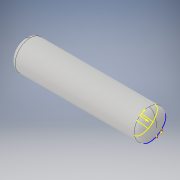
# Autodesk Inventor part: ModeloVaso
Saved by Autodesk Inventor 2019 (Build 230136000, 136)
## iProperties
Created: 2018-09-09
Part Number: ModeloVaso
Material: Generic
Document SubType Name: Modeling
Designer: leona
Density: 1 g/cm^3
Appearance: Default
Author: leona
Autodesk Inventor part; units mm, degrees
ref_plane "XZ Plane" through (0, 0, 0) normal (0, 1, 0) x (-1, 0, 0)
sketch "Sketch1" plane through (0, 0, 0) normal (0, 0, 1) x (1, 0, 0)
  line L0 (0, 50) -> (0, 0) construction
  line L1 (0, 0) -> (200, 0)
  line L2 (0, 50) -> (200, 50)
  ellipse E0 centre (200, 0) end of major axis (200, 50) minor radius 25 (225, 0) -> (200, 50) ccw
  line L3 (200, 0) -> (225, 0)
  line L4 (0, 50) -> (0, 0)
  line L5 (225, 0) -> (0, 0)
  dimension "d2" = 25
  dimension "d0" = 50
  dimension "d1" = 200
  constraints: 12 end point, 3 horizontal, 2 perpendicular, 1 coincident, 1 collinear, 1 point on line, 1 vertical, 4 other
  measures "d0" distance of L0.start L0.end
  measures "d1" distance of L0.end L1.end
revolve "Revolution1" add sketch "Sketch1" angle 360 about axis through (0, 0, 0) along (1, 0, 0)
mirror "Mirror1" about plane through (0, 50, 0) normal (-1, 0, 0) of "Revolution1"
ref_plane "Work Plane3" through (225, 0, 0) normal (1, 0, 0) x (0, 1, 0)
sketch "Sketch4" plane through (225, 0, 0) normal (1, 0, 0) x (0, 1, 0)
  line L0 (0, 0) -> (0, -20)
  line L1 (0, -20) -> (-1, -20)
  line L2 (1, -20) -> (0, -20)
  line L3 (1, -20) -> (0, -25)
  line L4 (0, -25) -> (-1, -20)
  line L5 (-20, 0) -> (-20, 1)
  line L6 (-20, -1) -> (-20, 0)
  line L7 (-20, -1) -> (-25, 0)
  line L8 (-25, 0) -> (-20, 1)
  line L9 (0, 0) -> (-20, 0)
  line L10 (0, 0) -> (50, 0) projected
  line L11 (-45.6527, 20.3919) -> (9.5558, -49.0784)
  circle A0 centre (0, 0) radius 50 projected
  line L12 (-18.0485, -14.3432) -> (0, 0)
  point P0 (-14.5002, -18.8081)
  point P1 (-26.6139, -3.5651)
  dimension "d6" = 1
  dimension "d13" = 5
  dimension "d14" = 20
  dimension "d17" = 90
  constraints: 24 end point, 4 point on line, 2 coincident, 2 collinear, 2 perpendicular, 2 point on circle, 1 midpoint, 1 vertical, 10 other
  measures "d6" distance of L0.end L1.end
  measures "d13" vertical distance of L2.start L3.end
  measures "d14" distance of L0.start L0.end
sketch3d "3D Sketch8"
ref_plane "Work Plane6" through (225, -18.0485, -14.3432) normal (0, 0.7829, 0.6222) x (-1, 0, 0)
sketch "Sketch6" plane through (225, -18.0485, -14.3432) normal (0, 0.7829, 0.6222) x (-1, 0, 0)
  line L0 (3.911, 13.7672) -> (25, 13.7672)
  line L1 (25, 13.7672) -> (3.911, 13.7672)
  line L2 (3, -5.7031) -> (25, -5.7031)
  point P0 (225, 0)
  point P1 (25, 44.3681)
  point P2 (25, -44.3681)
  point P3 (2.816, 0)
  constraints: 6 end point, 3 vertical alignment, 2 horizontal, 1 collinear, 1 other
ref_plane "Work Plane7" through (100, -39.1443, -31.1082) normal (0, 0.7829, 0.6222) x (-1, 0, 0)
sketch "Sketch7" plane through (100, -39.1443, -31.1082) normal (0, 0.7829, 0.6222) x (-1, 0, 0)
  spline S0 degree 3 poles (-100, 44.3681) (-101.4808, 44.3681) (-102.9197, 44.0717) (-105.9915, 42.8586) (-107.5313, 41.8403) (-111.1048, 38.7089) (-112.9353, 36.2558) (-117.1326, 29.0762) (-119.2485, 23.1879) (-121.1077, 13.9395) (-121.4968, 11.2864) (-121.9317, 6.9022) (-122.0507, 5.1608) (-122.1759, 1.9228) (-122.1957, 0.4216) (-122.1584, -2.647) (-122.0977, -4.2185) (-121.8605, -7.8257) (-121.654, -9.8674) (-120.8291, -15.7968) (-119.9952, -19.7203) (-117.0503, -29.1657) (-114.6544, -33.9776) (-110.0361, -39.7913) (-108.1121, -41.5075) (-105.1418, -43.2056) (-104.1316, -43.6442) (-102.0686, -44.2212) (-101.0421, -44.3681) (-100, -44.3681) knots 0 0 0 0 0.444236 0.444236 0.990273 0.990273 1.866665 1.866665 3.469962 3.469962 4.100671 4.100671 4.512916 4.512916 4.867731 4.867731 5.239347 5.239347 5.723479 5.723479 6.656656 6.656656 8.070297 8.070297 8.957642 8.957642 9.378299 9.378299 9.776887 9.776887 9.776887 9.776887 projected
  line L0 (-122, -5.7031) -> (-100, -5.7031) projected
  line L1 (-121.089, 13.7672) -> (-100, 13.7672) projected
  line L2 (-100, 50) -> (-100, -50) projected
  line L3 (-100, 0) -> (-115, 0)
  line L4 (-115, 0) -> (-115, 1)
  line L5 (-115, 1) -> (-118, 0)
  line L6 (-118, 0) -> (-115, -1)
  line L7 (-115, -1) -> (-115, 0)
  line L8 (-100, 0) -> (-100, -15)
  line L9 (-100, -15) -> (-101, -15)
  line L10 (-101, -15) -> (-100, -18)
  line L11 (-100, -18) -> (-99, -15)
  line L12 (-99, -15) -> (-100, -15)
  point P0 (100, 0)
  point P1 (-122.184, 0)
  point P2 (-100, -31.1082)
  dimension "d19" = 15
  dimension "d20" = 3
  dimension "d21" = 1
  dimension "d22" = 15
  dimension "d23" = 3
  dimension "d24" = 1
  constraints: 20 end point, 4 collinear, 3 point on line, 2 horizontal, 1 perpendicular, 4 other
  measures "d19" distance of L3.start L3.end
  measures "d20" horizontal distance of L5.end L6.end
  measures "d21" distance of L6.end L3.end
  measures "d22" distance of L3.start L8.end
  measures "d23" vertical distance of L10.end L11.end
  measures "d24" distance of L8.end L9.end
sketch3d "3D Sketch10"
body "Solid1"
